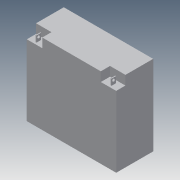
# Autodesk Inventor part: battery
Saved by Autodesk Inventor 2014 (Build 180170000, 170)
## iProperties
Created: 2016-01-12
Part Number: battery
Material: Generic
Document SubType Name: Modeling
Designer: Paul
Density: 1 g/cm^3
Appearance: Default
Author: Paul
Autodesk Inventor part; units mm, degrees
ref_plane "YZ Plane" through (0, 0, 0) normal (1, 0, 0) x (0, 1, 0)
ref_plane "XZ Plane" through (0, 0, 0) normal (0, 1, 0) x (-1, 0, 0)
ref_plane "XY Plane" through (0, 0, 0) normal (0, 0, 1) x (1, 0, 0)
sketch "Sketch1" plane through (0, 0, 0) normal (0, 0, 1) x (1, 0, 0)
  line L0 (0, 0) -> (184.15, 0)
  line L1 (184.15, 0) -> (184.15, 165.1)
  line L2 (184.15, 165.1) -> (0, 165.1)
  line L3 (0, 165.1) -> (0, 0)
  dimension "d0" = 184.15
  dimension "d1" = 165.1
  constraints: 8 end point, 2 parallel, 1 horizontal, 1 perpendicular
  measures "d0" distance of L2.end L1.end
  measures "d1" distance of L1.end L0.end
extrude "Extrusion1" add sketch "Sketch1" along normal blind 76.2
sketch "Sketch2" plane through (0, 0, 76.2) normal (0, 0, 1) x (1, 0, 0)
  line L0 (184.15, 165.1) -> (0, 165.1) projected
  line L1 (0, 165.1) -> (0, 0) projected
  line L2 (0, 165.1) -> (31.75, 165.1)
  line L3 (31.75, 165.1) -> (31.75, 146.05)
  line L4 (31.75, 146.05) -> (0, 146.05)
  line L5 (0, 146.05) -> (0, 165.1)
  line L6 (184.15, 165.1) -> (152.4, 165.1)
  line L7 (152.4, 165.1) -> (152.4, 146.05)
  line L8 (152.4, 146.05) -> (184.15, 146.05)
  line L9 (184.15, 146.05) -> (184.15, 165.1)
  dimension "d4" = 19.05
  dimension "d5" = 31.75
  constraints: 16 end point, 4 parallel, 2 collinear, 2 horizontal, 2 perpendicular
  measures "d4" distance between parallel lines of L4 L0
  measures "d5" distance between parallel lines of L3 L1
extrude "Extrusion2" cut sketch "Sketch2" against normal blind 19.05
sketch "Sketch3" plane through (152.4, 146.05, 76.2) normal (0, 1, 0) x (1, 0, 0)
  line L0 (-120.65, 0) -> (-152.4, 0) projected
  line L1 (-120.65, 0) -> (-120.65, 19.05) projected
  line L2 (-120.65, 19.05) -> (-152.4, 19.05) projected
  line L3 (-152.4, 0) -> (-152.4, 19.05) projected
  line L4 (-138.303, 13.6393) -> (-136.525, 13.6393)
  line L5 (-136.525, 13.6393) -> (-136.525, 4.1143)
  line L6 (-136.525, 4.1143) -> (-138.303, 4.1143)
  line L7 (-138.303, 4.1143) -> (-138.303, 13.6393)
  line L8 (-39.4488, 9.6539) -> (-37.1636, 9.6539)
  line L9 (-37.1636, 9.6539) -> (-37.1636, 4.1143)
  line L10 (-37.1636, 4.1143) -> (-39.4488, 4.1143)
  line L11 (-39.4488, 4.1143) -> (-39.4488, 9.6539)
  line L12 (16.0533, 4.1143) -> (17.8313, 4.1143)
  line L13 (17.8313, 4.1143) -> (17.8313, 13.6393)
  line L14 (17.8313, 13.6393) -> (16.0533, 13.6393)
  line L15 (16.0533, 13.6393) -> (16.0533, 4.1143)
  point P0 (-152.4, 76.2)
  dimension "d8" = 1.778
  dimension "d9" = 9.525
  constraints: 24 end point, 6 parallel, 3 collinear, 3 horizontal, 3 perpendicular
  measures "d8" distance of L5.end L6.end
  measures "d9" distance of L6.end L4.start
extrude "Extrusion3" add sketch "Sketch3" along normal blind 12.7 contours L4 L5 L6 L7 | L15 L14 L13 L12
sketch "Sketch4" plane through (170.2313, 146.05, 72.0857) normal (1, 0, 0) x (0, 0, -1)
  line L0 (0, 12.7) -> (9.525, 12.7) projected
  circle A0 centre (4.7625, 8.255) radius 3
  point P0 (72.0857, -146.05)
  dimension "d12" = 6
  dimension "d13" = 4.445
  constraints: 1 centre point
  measures "d12" diameter of A0
  measures "d13" distance from line of L0 A0.centre
extrude "Extrusion4" cut sketch "Sketch4" against normal blind 12.7
sketch "Sketch5" plane through (14.097, 146.05, 72.0857) normal (-1, 0, 0) x (0, 0, 1)
  line L0 (-9.525, 12.7) -> (0, 12.7) projected
  circle A0 centre (-4.7625, 8.255) radius 3
  point P0 (-72.0857, -146.05)
  dimension "d16" = 6
  dimension "d17" = 4.445
  constraints: 1 centre point
  measures "d16" diameter of A0
  measures "d17" distance from line of A0.centre L0
extrude "Extrusion5" cut sketch "Sketch5" against normal blind 12.7
body "Solid1"
